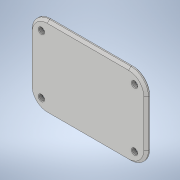
# Autodesk Inventor part: GPS_Antenna_FixV2
Saved by Autodesk Inventor 2021 (Build 250183000, 183)
## iProperties
Created: 2019-04-21
Part Number: GPS_Antenna_FixV2
Material: Generic
Document SubType Name: Modeling
Designer: lgnds
Density: 1 g/cm^3
Appearance: Default
Author: lgnds
## iProperties of the stored document _3DPrint.ipt
Created: 2021-02-19
Part Number: _3DPrint
Material: Generic
Document SubType Name: Modeling
Designer: Viktor
Density: 1 g/cm^3
Appearance: Default
Author: Viktor
Autodesk Inventor part; units mm, degrees
ref_plane "YZ Plane" through (0, 0, 0) normal (1, 0, 0) x (0, 1, 0)
ref_plane "XZ Plane" through (0, 0, 0) normal (0, 1, 0) x (-1, 0, 0)
ref_plane "XY Plane" through (0, 0, 0) normal (0, 0, 1) x (1, 0, 0)
sketch "Sketch1" plane through (0, 0, 0) normal (0, 0, 1) x (1, 0, 0)
  line L0 (-50, -35) -> (50, -35)
  line L1 (50, -35) -> (50, 35)
  line L2 (50, 35) -> (-50, 35)
  line L3 (-50, 35) -> (-50, -35)
  line L4 (-50, -35) -> (50, 35) construction
  line L5 (50, -35) -> (-50, 35) construction
  point P0 (0, 0)
  dimension "d0" = 100
  dimension "d1" = 70
  constraints: 12 end point, 2 midpoint, 2 parallel, 1 horizontal, 1 perpendicular
  measures "d0" distance of L1.end L2.end
  measures "d1" distance of L0.end L1.end
extrude "Extrusion1" add sketch "Sketch1" along normal blind 3.5
sketch "Sketch2" plane through (0, 0, 3.5) normal (0, 0, 1) x (1, 0, 0)
  circle A0 centre (-40, 25) radius 2.3
  line L0 (-70, 0) -> (70, 0) projected
  line L1 (0, -49) -> (0, 49) projected
  circle A1 centre (40, 25) radius 2.3
  circle A2 centre (-40, -25) radius 2.3
  circle A3 centre (40, -25) radius 2.3
  point P0 (0, 0)
  dimension "d4" = 40
  dimension "d5" = 25
  dimension "d6" = 4.6
  constraints: 4 centre point, 3 symmetric about line, 3 other
  measures "d4" distance from line of L1 A0.centre
  measures "d5" distance from line of L0 A0.centre
  measures "d6" diameter of A0
extrude "Extrusion2" cut sketch "Sketch2" against normal up to surface (3.5 mm away)
fillet "Fillet1" radius 15 4 edges at (-50, 35, 1.75) (-50, -35, 1.75) (50, -35, 1.75) (50, 35, 1.75)
chamfer "Chamfer2" distance 0.5 angle 45 12 edges at (-50, 0, 0) (-45.6066, -30.6066, 0) (0, -35, 0) (45.6066, -30.6066, 0) (50, 0, 0) (45.6066, 30.6066, 0) (0, 35, 0) (-45.6066, 30.6066, 0) (-42.3, -25, 0) (-42.3, 25, 0) (37.7, 25, 0) (37.7, -25, 0)
chamfer "Chamfer3" distance 0.5 angle 45 4 edges at (-42.3, 25, 3.5) (37.7, 25, 3.5) (37.7, -25, 3.5) (-42.3, -25, 3.5)
chamfer "Chamfer4" distance 2 angle 45 8 edges at (-50, 0, 3.5) (-45.6066, -30.6066, 3.5) (0, -35, 3.5) (45.6066, -30.6066, 3.5) (50, 0, 3.5) (45.6066, 30.6066, 3.5) (0, 35, 3.5) (-45.6066, 30.6066, 3.5)
body "Solid1"
